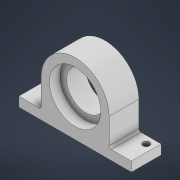
# Autodesk Inventor part: Halterung_Differential_3
Saved by Autodesk Inventor 2021 (Build 250183000, 183)
## iProperties
Created: 2021-01-24
Part Number: Halterung_Differential_3
Material: Generisch
Document SubType Name: Modeling
Designer: Ctroi
Density: 1 g/cm^3
Appearance: Vorgabe
Author: Ctroi
Autodesk Inventor part; units mm, degrees
ref_plane "YZ Plane" through (0, 0, 0) normal (1, 0, 0) x (0, 1, 0)
ref_plane "XZ Plane" through (0, 0, 0) normal (0, 1, 0) x (-1, 0, 0)
ref_plane "XY Plane" through (0, 0, 0) normal (0, 0, 1) x (1, 0, 0)
sketch "Skizze1" plane through (0, 0, 0) normal (0, 0, 1) x (1, 0, 0)
  line L0 (0, 22.4) -> (0, -22.4) projected
  line L1 (-22.4, 0) -> (22.4, 0) projected
  line L2 (-16, 16) -> (16, 16)
  line L3 (16, 16) -> (16, -16)
  line L4 (16, -16) -> (-16, -16)
  line L5 (-16, -16) -> (-16, 16)
  circle A0 centre (0, 0) radius 12.1
  dimension "d0" = 32
  dimension "d1" = 32
  dimension "d2" = 24.2
  constraints: 8 end point, 2 parallel, 1 centre point, 1 coincident, 1 horizontal, 1 perpendicular, 2 other
  measures "d0" distance of L3.end L4.end
  measures "d1" distance of L2.end L3.end
  measures "d2" diameter of A0
extrude "Extrusion1" add sketch "Skizze1" along normal blind 14 contours L2 L3 L1 A0 L0 | L0 A0 L1 L5 L2 | L1 L3 L4 L0 A0 | A0 L0 L4 L5 L1
sketch "Skizze2" plane through (16, -16, 0) normal (1, 0, 0) x (0, 0, -1)
  line L0 (-14, 32) -> (-14, 0) projected
  line L1 (0, 32) -> (0, 0) projected
  line L2 (-14, 0) -> (0, 0)
  line L3 (0, 0) -> (0, 3)
  line L4 (0, 3) -> (-14, 3)
  line L5 (-14, 3) -> (-14, 0)
  point P0 (0, 16)
  point P1 (-14, 3)
  dimension "d5" = 3
  constraints: 8 end point, 2 parallel, 1 horizontal, 1 perpendicular, 1 point on line
  measures "d5" distance of L3.end L2.end
sketch "Skizze3" plane through (-16, -16, 0) normal (-1, 0, 0) x (0, 0, 1)
  line L0 (14, 32) -> (14, 0) projected
  line L1 (0, 32) -> (0, 0) projected
  line L2 (14, 0) -> (0, 0)
  line L3 (0, 0) -> (0, 3)
  line L4 (0, 3) -> (14, 3)
  line L5 (14, 3) -> (14, 0)
  point P0 (0, 16)
  point P1 (14, 3)
  dimension "d6" = 3
  constraints: 8 end point, 2 parallel, 1 horizontal, 1 perpendicular, 1 point on line
  measures "d6" distance of L2.end L3.end
extrude "Extrusion2" add sketch "Skizze3" along normal blind 10.5
extrude "Extrusion3" add sketch "Skizze2" along normal blind 10.5
sketch "Skizze4" plane through (0, 0, 0) normal (0, 0, -1) x (-1, 0, 0)
  circle A0 centre (0, 0) radius 12.1
  circle A1 centre (0, 0) radius 12.1 projected
  circle A2 centre (0, 0) radius 9
  dimension "d11" = 24.2
  dimension "d12" = 18
  constraints: 2 centre point, 2 coincident
  measures "d11" diameter of A0
  measures "d12" diameter of A2
extrude "Extrusion4" add sketch "Skizze4" against normal blind 9
fillet "Rundung1" radius 16 2 edges at (16, 16, 7) (-16, 16, 7)
sketch "Skizze5" plane through (16, -13, 14) normal (0, 1, 0) x (1, 0, 0)
  circle A0 centre (-39, 10.5) radius 1.6
  line L0 (-32, 14) -> (-42.5, 14) projected
  line L1 (-42.5, 0) -> (-42.5, 14) projected
  circle A1 centre (7, 10.5) radius 1.6
  line L2 (0, 14) -> (10.5, 14) projected
  line L3 (10.5, 14) -> (10.5, 0) projected
  point P0 (-16, 14)
  dimension "d16" = 3.2
  dimension "d17" = 3.5
  dimension "d18" = 3.5
  dimension "d19" = 3.2
  dimension "d20" = 3.5
  dimension "d21" = 3.5
  constraints: 2 centre point
  measures "d16" diameter of A0
  measures "d17" distance from line of L0 A0.centre
  measures "d18" distance from line of L1 A0.centre
  measures "d19" diameter of A1
  measures "d20" distance from line of L2 A1.centre
  measures "d21" distance from line of L3 A1.centre
extrude "Extrusion5" cut sketch "Skizze5" against normal up to surface (3 mm away)
fillet "Rundung2" radius 1 2 edges at (-16, -13, 7) (16, -13, 7)
sketch "Skizze6" plane through (-26.5, -16, 0) normal (0, -1, 0) x (1, 0, 0)
  line L0 (53, 14) -> (0, 14) projected
  line L1 (53, 14) -> (53, 0) projected
  line L2 (0, 14) -> (53, 14)
  line L3 (53, 14) -> (53, 0)
  line L4 (53, 0) -> (0, 0)
  line L5 (0, 0) -> (0, 14)
  circle A0 centre (3.5, 3.5) radius 1.6 projected
  circle A1 centre (3.5, 3.5) radius 1.6
  circle A2 centre (49.5, 3.5) radius 1.6 projected
  circle A3 centre (49.5, 3.5) radius 1.6
  point P0 (26.5, 0)
  dimension "d25" = 3.2
  dimension "d26" = 3.2
  constraints: 8 end point, 2 centre point, 2 coincident, 2 parallel, 1 horizontal, 1 perpendicular
  measures "d25" diameter of A3
  measures "d26" diameter of A1
extrude "Extrusion6" add sketch "Skizze6" along normal blind 1.5
